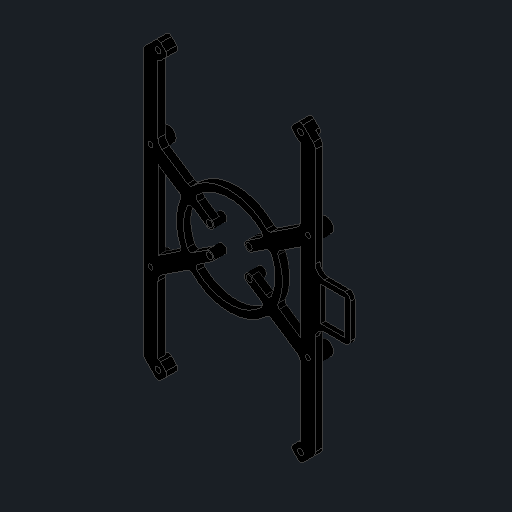
# Autodesk Inventor part: Center Hub
Saved by Autodesk Inventor 2026.1 (Build 301233020, 233B)
## iProperties
Created: 2025-12-12
Part Number: Center Hub
Material: Generic
Document SubType Name: Modeling
Designer: Bahaa
Density: 1 g/cm^3
Appearance: Default
Author: Bahaa
Autodesk Inventor part; units mm, degrees
ref_plane "YZ Plane" through (0, 0, 0) normal (1, 0, 0) x (0, 1, 0)
ref_plane "XZ Plane" through (0, 0, 0) normal (0, 1, 0) x (-1, 0, 0)
ref_plane "XY Plane" through (0, 0, 0) normal (0, 0, 1) x (1, 0, 0)
sketch "Sketch1" plane through (0, 0, 0) normal (0, 1, 0) x (-1, 0, 0)
  line L0 (-38.8909, 75.6604) -> (38.8909, 75.6604) construction
  line L1 (38.8909, 75.6604) -> (38.8909, -75.6604) construction
  line L2 (38.8909, -75.6604) -> (-38.8909, -75.6604) construction
  line L3 (-38.8909, -75.6604) -> (-38.8909, 75.6604) construction
  line L4 (38.8909, 81.3173) -> (33.234, 75.6604)
  line L5 (33.234, 75.6604) -> (38.8909, 70.0036)
  line L6 (38.8909, 70.0036) -> (44.5477, 75.6604)
  line L7 (44.5477, 75.6604) -> (38.8909, 81.3173)
  line L8 (38.8909, 81.3173) -> (38.8909, 70.0036) construction
  line L9 (33.234, 75.6604) -> (44.5477, 75.6604) construction
  line L10 (38.8909, 81.3173) -> (46.8909, 81.3173) construction
  line L11 (43, 29) -> (-43, 29) construction
  line L12 (-43, 29) -> (-43, -29) construction
  line L13 (-43, -29) -> (43, -29) construction
  line L14 (43, -29) -> (43, 29) construction
  line L15 (43, 29) -> (-43, -29) construction
  line L16 (-43, 29) -> (43, -29) construction
  circle A0 centre (43, 29) radius 4
  line L17 (38.8909, 75.6604) -> (43, 71.5513) construction
  line L18 (43, 71.5513) -> (43, 29) construction
  line L19 (36.0625, 72.832) -> (39, 69.8945)
  line L20 (39, 69.8945) -> (39, 29)
  line L21 (41.7193, 78.4889) -> (47, 73.2082)
  line L22 (47, 73.2082) -> (47, 29)
  line L23 (-10.795, -7.62) -> (10.795, -7.62) construction
  line L24 (10.795, -7.62) -> (10.795, 7.62) construction
  line L25 (10.795, 7.62) -> (-10.795, 7.62) construction
  line L26 (-10.795, 7.62) -> (-10.795, -7.62) construction
  line L27 (-10.795, -7.62) -> (10.795, 7.62) construction
  line L28 (10.795, -7.62) -> (-10.795, 7.62) construction
  line L29 (43, 0) -> (0, 0) construction
  line L30 (0, 0) -> (0, 29) construction
  line L31 (38.8909, -81.3173) -> (33.234, -75.6604)
  line L32 (33.234, -75.6604) -> (38.8909, -70.0036)
  line L33 (44.5477, -75.6604) -> (38.8909, -81.3173)
  circle A1 centre (43, -29) radius 4
  line L34 (36.0625, -72.832) -> (39, -69.8945)
  line L35 (39, -69.8945) -> (39, -29)
  line L36 (41.7193, -78.4889) -> (47, -73.2082)
  line L37 (47, -73.2082) -> (47, -29)
  line L38 (-38.8909, 81.3173) -> (-33.234, 75.6604)
  line L39 (-33.234, 75.6604) -> (-38.8909, 70.0036)
  line L40 (-44.5477, 75.6604) -> (-38.8909, 81.3173)
  circle A2 centre (-43, 29) radius 4
  line L41 (-36.0625, 72.832) -> (-39, 69.8945)
  line L42 (-39, 69.8945) -> (-39, 29)
  line L43 (-41.7193, 78.4889) -> (-47, 73.2082)
  line L44 (-47, 73.2082) -> (-47, 29)
  line L45 (-36.0625, -72.832) -> (-39, -69.8945)
  line L46 (-39, -69.8945) -> (-39, -29)
  line L47 (-38.8909, -81.3173) -> (-33.234, -75.6604)
  line L48 (-44.5477, -75.6604) -> (-38.8909, -81.3173)
  line L49 (-33.234, -75.6604) -> (-38.8909, -70.0036)
  line L50 (-41.7193, -78.4889) -> (-47, -73.2082)
  line L51 (-47, -73.2082) -> (-47, -29)
  circle A3 centre (-43, -29) radius 4
  line L52 (43, 29) -> (10.795, 7.62) construction
  line L53 (40.7877, 32.3325) -> (8.5827, 10.9525)
  line L54 (13.0073, 4.2875) -> (45.2123, 25.6675)
  arc A4 (45.2123, 25.6675) -> (40.7877, 32.3325) centre (43, 29) ccw
  arc A5 (8.5827, 10.9525) -> (13.0073, 4.2875) centre (10.795, 7.62) ccw
  line L55 (43, -29) -> (10.795, -7.62) construction
  line L56 (45.2123, -25.6675) -> (13.0073, -4.2875)
  line L57 (8.5827, -10.9525) -> (40.7877, -32.3325)
  arc A6 (40.7877, -32.3325) -> (45.2123, -25.6675) centre (43, -29) ccw
  arc A7 (13.0073, -4.2875) -> (8.5827, -10.9525) centre (10.795, -7.62) ccw
  line L58 (-43, 29) -> (-10.795, 7.62) construction
  line L59 (-45.2123, 25.6675) -> (-13.0073, 4.2875)
  line L60 (-8.5827, 10.9525) -> (-40.7877, 32.3325)
  arc A8 (-40.7877, 32.3325) -> (-45.2123, 25.6675) centre (-43, 29) ccw
  arc A9 (-13.0073, 4.2875) -> (-8.5827, 10.9525) centre (-10.795, 7.62) ccw
  line L61 (-43, -29) -> (-10.795, -7.62) construction
  line L62 (-40.7877, -32.3325) -> (-8.5827, -10.9525)
  line L63 (-13.0073, -4.2875) -> (-45.2123, -25.6675)
  arc A10 (-45.2123, -25.6675) -> (-40.7877, -32.3325) centre (-43, -29) ccw
  arc A11 (-8.5827, -10.9525) -> (-13.0073, -4.2875) centre (-10.795, -7.62) ccw
  line L64 (38.8909, -70.0036) -> (44.5477, -75.6604)
  line L65 (-38.8909, 70.0036) -> (-44.5477, 75.6604)
  line L66 (-38.8909, -70.0036) -> (-44.5477, -75.6604)
  line L67 (39, 69.8945) -> (44.6569, 75.5513)
  line L68 (39, -69.8945) -> (44.6569, -75.5513)
  line L69 (-39, -69.8945) -> (-44.6569, -75.5513)
  line L70 (-39, 69.8945) -> (-44.6569, 75.5513)
  circle A12 centre (0, 0) radius 29
  circle A13 centre (0, 0) radius 25
  line L71 (23.9496, 16.3529) -> (10.795, 7.62) construction
  line L72 (22.5668, 18.4358) -> (9.4123, 9.7028)
  line L73 (12.1777, 5.5372) -> (25.3323, 14.2701)
  arc A14 (25.3323, 14.2701) -> (22.5668, 18.4358) centre (23.9496, 16.3529) ccw
  arc A15 (9.4123, 9.7028) -> (12.1777, 5.5372) centre (10.795, 7.62) ccw
  line L74 (10.795, -7.62) -> (23.9496, -16.3529) construction
  line L75 (9.4123, -9.7028) -> (22.5668, -18.4358)
  line L76 (25.3323, -14.2701) -> (12.1777, -5.5372)
  arc A16 (12.1777, -5.5372) -> (9.4123, -9.7028) centre (10.795, -7.62) ccw
  arc A17 (22.5668, -18.4358) -> (25.3323, -14.2701) centre (23.9496, -16.3529) ccw
  line L77 (-10.795, 7.62) -> (-23.9496, 16.3529) construction
  line L78 (-9.4123, 9.7028) -> (-22.5668, 18.4358)
  line L79 (-25.3323, 14.2701) -> (-12.1777, 5.5372)
  arc A18 (-12.1777, 5.5372) -> (-9.4123, 9.7028) centre (-10.795, 7.62) ccw
  arc A19 (-22.5668, 18.4358) -> (-25.3323, 14.2701) centre (-23.9496, 16.3529) ccw
  line L80 (-10.795, -7.62) -> (-23.9496, -16.3529) construction
  line L81 (-12.1777, -5.5372) -> (-25.3323, -14.2701)
  line L82 (-22.5668, -18.4358) -> (-9.4123, -9.7028)
  arc A20 (-9.4123, -9.7028) -> (-12.1777, -5.5372) centre (-10.795, -7.62) ccw
  arc A21 (-25.3323, -14.2701) -> (-22.5668, -18.4358) centre (-23.9496, -16.3529) ccw
  line L83 (-21.9267, 12.0092) -> (-24.6387, 12.0092)
  line L84 (-21.9267, -12.0092) -> (-24.6387, -12.0092)
  circle A22 centre (-10.795, 7.62) radius 2.5
  circle A23 centre (-10.795, -7.62) radius 2.5
  circle A24 centre (43, 71.5513) radius 4
  circle A25 centre (43, -71.5513) radius 4
  circle A26 centre (-43, 71.5513) radius 4
  circle A27 centre (-43, -71.5513) radius 4
  line L85 (-47, 29) -> (-47, 26.8543)
  line L86 (-47, 26.8543) -> (-45.2123, 25.6675)
  line L87 (-47, -29) -> (-47, -26.8543)
  line L88 (-47, -26.8543) -> (-45.2123, -25.6675)
  line L89 (47, 29) -> (47, 26.8543)
  line L90 (47, 26.8543) -> (45.2123, 25.6675)
  line L91 (47, -29) -> (47, -26.8543)
  line L92 (47, -26.8543) -> (45.2123, -25.6675)
  circle A28 centre (10.795, 7.62) radius 2.5
  circle A29 centre (10.795, -7.62) radius 2.5
  line L93 (47, 26.8543) -> (43.0003, 29.0002)
  line L94 (47, 26.8543) -> (38.8909, 26.8543)
  line L95 (38.8909, 26.8543) -> (38.8909, -26.8543)
  line L96 (38.8909, -26.8543) -> (47, -26.8543)
  line L97 (47, -26.8543) -> (47, 26.8543)
  line L98 (-38.8909, 26.8543) -> (-38.8909, -26.8543)
  line L99 (-47, -26.8543) -> (-47, 26.8543)
  line L100 (-47, 0) -> (-66.2, 0) construction
  line L101 (-63.2, 9.35) -> (-50, 9.35)
  line L102 (-50, 9.35) -> (-50, -9.35)
  line L103 (-50, -9.35) -> (-63.2, -9.35)
  line L104 (-63.2, -9.35) -> (-63.2, 9.35)
  line L105 (-63.2, 9.35) -> (-50, -9.35) construction
  line L106 (-50, 9.35) -> (-63.2, -9.35) construction
  line L107 (-47, -12.35) -> (-47, 12.35)
  line L108 (-47, 12.35) -> (-66.2, 12.35)
  line L109 (-66.2, 12.35) -> (-66.2, -12.35)
  line L110 (-66.2, -12.35) -> (-47, -12.35)
  point P0 (0, 75.6604)
  point P1 (-10.795, 0)
  point P2 (26.8975, 18.31)
  point P3 (26.8975, -18.31)
  point P4 (-26.8975, 18.31)
  point P5 (-26.8975, -18.31)
  point P6 (45.2123, -25.6675)
  point P7 (39, -31.1457)
  point P8 (-39, -31.1457)
  point P9 (-45.2123, -25.6675)
  point P10 (-39, 31.1457)
  point P11 (47, 29)
  point P12 (39, 31.1457)
  point P13 (-40.7877, -32.3325)
  point P14 (-39, -29)
  point P15 (-44.5477, -75.6604)
  point P16 (-39, 29)
  point P17 (-44.5477, 75.6604)
  point P18 (40.7877, 32.3325)
  point P19 (17.3723, 11.9865)
  point P20 (17.3723, -11.9865)
  point P21 (-17.3723, 11.9865)
  point P22 (-17.3723, -11.9865)
  point P23 (19.0979, 16.1328)
  point P24 (21.9267, 12.0092)
  point P25 (21.9267, -12.0092)
  point P26 (19.0979, -16.1328)
  point P27 (-19.0979, -16.1328)
  point P28 (-21.6814, -12.4466)
  point P29 (-22.6117, -10.6636)
  point P30 (-21.4624, -19.503)
  point P31 (21.4624, -19.503)
  point P32 (25.9748, -12.8962)
  point P33 (25.9748, 12.8962)
  point P34 (21.4624, 19.503)
  point P35 (-21.4624, 19.503)
  point P36 (-22.6117, 10.6636)
  point P37 (-21.6814, 12.4466)
  point P38 (-19.0979, 16.1328)
  point P39 (-12.1777, -5.5372)
  point P40 (-12.1777, 5.5372)
  point P41 (47, 71.5513)
  point P42 (45.8284, 74.3797)
  point P43 (-47, 71.5513)
  point P44 (-45.8284, 74.3797)
  point P45 (-47, -71.5513)
  point P46 (-45.8284, -74.3797)
  point P47 (45.8284, -74.3797)
  point P48 (47, -71.5513)
  point P49 (47, 29)
  point P50 (-25.9748, 12.8962)
  point P51 (-25.9748, -12.8962)
  point P52 (38.8909, 21.4709)
  point P53 (38.8909, -21.4709)
  point P54 (-56.6, 0)
  point P55 (-38.8909, -21.4709)
  point P56 (-38.8909, 21.4709)
  dimension "d1" = 77.7818
  dimension "d2" = 151.3209
  dimension "d3" = 38.8909
  dimension "d4" = 75.6604
  dimension "d5" = 38.8909
  dimension "d6" = 75.6604
  dimension "d7" = 8
  dimension "d8" = 135
  dimension "d9" = 8
  dimension "d10" = 86
  dimension "d11" = 58
  dimension "d12" = 8
  dimension "d13" = 4.1091
  dimension "d14" = 4
  dimension "d15" = 4
  dimension "d17" = 7.62
  dimension "d19" = 10.795
  dimension "d20" = 21.59
  dimension "d21" = 15.24
  dimension "d22" = 8
  dimension "d23" = 8
  dimension "d24" = 8
  dimension "d25" = 8
  dimension "d30" = 58
  dimension "d31" = 50
  dimension "d32" = 5
  dimension "d33" = 5
  dimension "d34" = 5
  dimension "d35" = 5
  dimension "d66" = 4.539
  dimension "d85" = 19.2
  dimension "d86" = 13.2
  dimension "d87" = 18.7
  dimension "d88" = 3
  constraints: 238 end point, 45 symmetric about line, 38 point on circle, 34 tangent, 25 centre point, 22 midpoint, 22 parallel, 14 point on line, 11 perpendicular, 9 horizontal, 7 coincident, 2 vertical, 1 collinear, 1 equal length, 26 other
  measures "d1" distance of L1.end L2.end
  measures "d2" distance of L0.end L1.end
  measures "d3" distance from line of L3 point (0, 0)
  measures "d4" distance of point (0, 75.66) point (0, 0)
  measures "d5" distance from line of point (0, 0) L1
  measures "d6" distance from line of point (0, 0) L0
  measures "d7" distance of L4.start L4.end
  measures "d8" angle of L4 L10
  measures "d9" distance of L5.end L4.end
  measures "d10" distance of L13.end L12.end
  measures "d11" distance of L12.end L11.end
  measures "d12" diameter of A0
  measures "d13" horizontal distance of L0.end L17.end
  measures "d14" distance between parallel lines of L17 L19
  measures "d15" distance between parallel lines of L17 L21
  measures "d17" distance from line of L23 point (0, 0)
  measures "d19" distance of point (-10.795, 0) point (0, 0)
  measures "d20" distance of L23.start L23.end
  measures "d21" distance of L23.end L24.end
  measures "d22" diameter of A5
  measures "d23" diameter of A7
  measures "d24" diameter of A9
  measures "d25" diameter of A11
  measures "d30" diameter of A12
  measures "d31" diameter of A13
  measures "d32" diameter of A15
  measures "d33" diameter of A17
  measures "d34" diameter of A19
  measures "d35" diameter of A21
  measures "d66" distance of L90.start L93.end
  measures "d85" distance of L100.start L100.end
  measures "d86" distance of L102.end L103.end
  measures "d87" distance of L101.end L102.end
  measures "d88" distance between parallel lines of L102 L107
extrude "Extrusion1" add sketch "Sketch1" along normal blind 4 contours L7 L6 A24 L5 L4 | L21 L67 A24 L6 | L6 A24 L67 L19 | A24 L67 L6 | L6 A24 | L21 A24 L67 | L67 A24 L22 A0 L53 L20 | A24 L67 | L53 A0 L20 | L20 A0 L94 L95 L54 A12 L73 A14 L72 L53 | A0 L94 | A12 L72 A13 L53 | L53 A13 L60 A12 | L89 L93 A0 | L94 A0 | A0 L54 L95 L94 | L72 A14 L73 A12 | A12 L73 A13 L72 | A12 L78 A19 L79 L59 A2 L42 L60 | L60 A13 L78 A12 | L93 L94 A0 | L97 L92 L56 L95 L54 L90 | L90 A0 L94 | A13 L73 A28 L72 | A12 L54 A13 L73 | L60 A2 L44 A26 L70 L42 | L42 A2 L60 | L78 A13 L79 A12 | A12 L79 A19 L78 | L96 A1 L92 | L91 A1 L96 | A28 A15 | L78 A22 L79 A13 | A12 L56 A13 L54 | L70 A26 L65 L41 | A2 | L79 L83 L59 A12 | L37 A25 L68 L35 L57 A1 | A1 L96 | A1 L96 | A1 L96 L95 L56 | L95 L96 A1 L35 L57 A12 L75 A17 L76 L56 | A13 L59 L83 | A18 A22 | L65 A26 L40 L38 L39 | A26 L70 | L70 A26 L65 | L86 L85 A2 | L59 L98 L63 L88 L99 L86 | L59 A13 L63 A12 | L57 L35 A1 | A25 L68 | A12 L76 A13 L56 | L65 A26 | A26 L43 L70 | L70 L43 L65 A26 | A12 L81 A21 L82 L62 L46 A3 L63 | L63 L84 L81 A12 | A25 L64 L34 L68 | L68 A25 L64 | L36 L68 A25 | L76 A17 L75 A12 | A12 L75 A13 L76 | A13 L84 L63 | L81 A13 L82 A12 | A12 L82 A21 L81 | A12 L62 A13 L57 | L57 A13 L75 A12 | L68 L36 L64 A25 | A25 L64 L33 L31 L32 | L64 A25 | A13 L75 A29 L76 | L81 A23 L82 A13 | A3 | A3 L87 L88 | L82 A13 L62 A12 | A29 A16 | A20 A23 | L46 L62 A3 | A3 L62 L46 L69 A27 L51 | A27 L69 | L45 L66 A27 L69 | A27 L66 L69 | A27 L69 L50 | L45 L49 L47 L48 L66 A27 | A27 L66 L50 L69 | A27 L66
extrude "Extrusion2" add sketch "Sketch1" along normal blind 6 contours L7 L6 A24 L5 L4 | L21 L67 A24 L6 | L6 A24 L67 L19 | A24 L67 L6 | L6 A24 | L70 A26 L65 L41 | L65 A26 L40 L38 L39 | L70 A26 L65 | L65 A26 | L70 L43 L65 A26 | A25 L64 L34 L68 | L68 A25 L64 | L68 L36 L64 A25 | A25 L64 L33 L31 L32 | L64 A25 | L45 L66 A27 L69 | A27 L66 L69 | L45 L49 L47 L48 L66 A27 | A27 L66 L50 L69 | A27 L66
extrude "Extrusion3" add sketch "Sketch1" along normal blind 7 contours A28 A15 | A18 A22 | A29 A16 | A20 A23
fillet "Fillet1" [suppressed]
fillet "Fillet2" radius 2 32 edges at (-19.0979, 2, 16.1328) (-21.9267, 2, 12.0092) (-21.9267, 2, -12.0092) (-19.0979, 2, -16.1328) (19.0979, 2, 16.1328) (19.0979, 2, -16.1328) (-21.4624, 2, 19.503) (-25.9748, 2, 12.8962) (-21.4624, 2, -19.503) (-25.9748, 2, -12.8962) (21.4624, 2, -19.503) (21.4624, 2, 19.503) (-33.234, 3, 75.6604) (-38.8909, 3, 81.3173) (-39, 5, 69.8945) (-44.6569, 5, 75.5513) (44.6569, 5, 75.5513) (39, 5, 69.8945) (38.8909, 3, 81.3173) (33.234, 3, 75.6604) (44.6569, 5, -75.5513) (39, 5, -69.8945) (33.234, 3, -75.6604) (38.8909, 3, -81.3173) (-33.234, 3, -75.6604) (-39, 5, -69.8945) (-38.8909, 3, -81.3173) (-44.6569, 5, -75.5513) (25.9748, 2, 12.8962) (25.9748, 2, -12.8962) (21.9267, 2, 12.0092) (21.9267, 2, -12.0092)
fillet "Fillet3" radius 5 4 edges at (-39, 2, 31.1457) (-39, 2, -31.1457) (39, 2, -31.1457) (39, 2, 31.1457)
sketch "Sketch2" plane through (0, 7, 0) normal (0, 1, 0) x (1, 0, 0)
  line L0 (-43.2426, -74.1371) -> (-40.4142, -71.3087) projected
  line L1 (-37.4767, -79.9031) -> (-34.6482, -77.0746) projected
  line L2 (-34.6482, -74.2462) -> (-37.5858, -71.3087) projected
  line L3 (0, 0) -> (-25, 0) construction
  arc A0 (-22.969, 9.8704) -> (-22.969, -9.8704) centre (0, 0) ccw construction
  line L4 (0, 0) -> (0, 25) construction
  line L5 (43.2426, -74.1371) -> (40.4142, -71.3087)
  line L6 (37.4767, -79.9031) -> (34.6482, -77.0746)
  line L7 (34.6482, -74.2462) -> (37.5858, -71.3087)
  circle A1 centre (10.795, 7.62) radius 2.5 projected
  point P0 (-38.8909, -75.6604)
  point P1 (-41.8284, -72.7229)
  point P2 (-38.8909, 75.6604)
  point P3 (38.8909, -75.6604)
  point P4 (41.8284, -72.7229)
  point P5 (38.8909, 75.6604)
  dimension "d74" = 151.3209
  dimension "d75" = 77.7818
  constraints: 10 end point, 10 symmetric about line, 1 horizontal, 1 midpoint, 1 point on circle, 1 vertical
  measures "d74" diameter of point (-38.891, 75.66) L3
  measures "d75" distance of point (38.891, 75.66) point (-38.891, 75.66)
hole "Hole1" at (-38.8909, 7, 75.6604) at (-38.8909, 7, -75.6604) at (38.8909, 7, 75.6604) at (38.8909, 7, -75.6604) direction (0, -1, 0) diameter 3.2 end through all counterbore diameter 5.7 counterbore depth 3
sketch "Sketch3" plane through (-10.795, 0, 7.62) normal (0, 1, 0) x (1, 0, 0)
  circle A0 centre (0, 0) radius 2.5 projected
  circle A1 centre (0, 15.24) radius 2.5 projected
  circle A2 centre (21.59, 15.24) radius 2.5 projected
  circle A3 centre (21.59, 0) radius 2.5 projected
  point P0 (10.795, 7.62)
  point P1 (-32.205, -21.38)
  point P2 (-32.205, 36.62)
  point P3 (53.795, -21.38)
  point P4 (53.795, 36.62)
hole "Hole3" at (-10.795, 0, 7.62) at (-10.795, 0, -7.62) at (10.795, 0, 7.62) at (10.795, 0, -7.62) direction (0, 1, 0) diameter 3.4 depth 5.7
extrude "Extrusion4" add sketch "Sketch1" along normal blind 6 from surface at 4 contours A0 L94 | L94 A0 | A2 | A1 L96 | A1 L96 | A3
sketch "Sketch5" plane through (-43, 10, 29) normal (0, 1, 0) x (1, 0, 0)
  circle A0 centre (0, 0) radius 4 projected
  circle A1 centre (0, 58) radius 4 projected
  circle A2 centre (86, 0) radius 4 projected
  circle A3 centre (86, 58) radius 4 projected
  point P0 (43, 29)
hole "Hole5" at (-43, 10, 29) at (-43, 10, -29) at (43, 10, 29) at (43, 10, -29) direction (0, -1, 0) diameter 2.7 end through all
extrude "Extrusion5" add sketch "Sketch1" along normal blind 2.5 contours L99 L110 L109 L108
fillet "Fillet4" radius 3 2 edges at (66.2, 1.25, 12.35) (66.2, 1.25, -12.35)
fillet "Fillet5" radius 5 2 edges at (47, 1.25, 12.35) (47, 1.25, -12.35)
equation "\"d3\" = 0.5 * d1"
equation "\"d4\" = 0.5 * d2"
equation "\"d5\" = 0.5 * d1"
equation "\"d6\" = 0.5 * d2"
equation "\"d9\" = d7"
equation "\"d12\" = d7"
equation "\"d14\" = 0.5 * d7"
equation "\"d15\" = 0.5 * d7"
equation "\"d20\" = 2 * d19"
equation "\"d21\" = 2 * d17"
equation "\"d23\" = d22"
equation "\"d24\" = d22"
equation "\"d25\" = d22"
body "Solid1"
